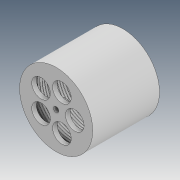
# Autodesk Inventor part: PeepCover
Saved by Autodesk Inventor 2020 (Build 240168000, 168)
## iProperties
Created: 2020-04-09
Part Number: PeepCover
Material: Generic
Document SubType Name: Modeling
Designer: Theo Cominotto
Density: 1 g/cm^3
Appearance: Default
Author: Theo Cominotto
Autodesk Inventor part; units mm, degrees
ref_plane "YZ Plane" through (0, 0, 0) normal (1, 0, 0) x (0, 1, 0)
ref_plane "XZ Plane" through (0, 0, 0) normal (0, 1, 0) x (-1, 0, 0)
ref_plane "XY Plane" through (0, 0, 0) normal (0, 0, 1) x (1, 0, 0)
sketch "Sketch1" plane through (0, 0, 0) normal (0, 0, 1) x (1, 0, 0)
  circle A0 centre (0, 0) radius 21.95
  circle A1 centre (0, 0) radius 23.55
  dimension "d0" = 43.9
  dimension "d1" = 1.6
  constraints: 2 centre point, 1 coincident
  measures "d0" diameter of A0
  measures "d1" radial gap between concentric circles of A0 A1
extrude "Extrusion1" add sketch "Sketch1" along normal blind 40
sketch "Sketch2" plane through (0, 0, 0) normal (0, 1, 0) x (-1, 0, 0)
  line L0 (23.55, 0) -> (-23.55, 0) projected
  line L1 (23.55, 0) -> (23.55, -1.2)
  line L2 (23.55, -0.6) -> (24.35, -0.6) construction
  line L3 (24.35, -0.6) -> (23.55, -1.2)
  line L4 (24.35, -0.6) -> (23.55, 0)
  line L5 (23.55, 0) -> (21.95, 0) construction
  line L6 (21.95, 40) -> (21.95, 0) construction
  line L7 (22.75, 0) -> (22.75, -1.2) construction
  line L8 (21.95, 0) -> (21.95, -1.2)
  line L9 (21.95, -0.6) -> (21.15, -0.6) construction
  line L10 (21.15, -0.6) -> (21.95, -1.2)
  line L11 (21.15, -0.6) -> (21.95, 0)
  point P0 (0, 0)
  dimension "d4" = 1.2
  dimension "d5" = 0.8
  constraints: 20 end point, 3 symmetric about line, 2 midpoint, 2 point on line, 2 vertical, 1 horizontal
  measures "d4" distance of L0.start L1.end
  measures "d5" distance of L2.start L2.end
coil "Coil1" sketch "Sketch2" operation add axis through (0, 0, -10) along (0, 0, 1) pitch 1.5 turns 26.666667 hand right contours L8 L10 L11
sketch "Sketch3" plane through (0, 0, 0) normal (0, 0, -1) x (-1, 0, 0)
  circle A0 centre (0, 0) radius 23.55 projected
extrude "Extrusion2" cut sketch "Sketch3" along normal blind 20
sketch "Sketch4" plane through (0, 0, 40) normal (0, 0, 1) x (1, 0, 0)
  circle A0 centre (0, 0) radius 23.55 projected
  line L0 (0, 0) -> (12, 0) construction
  circle A1 centre (12, 0) radius 6
  circle A2 centre (3.7082, 11.4127) radius 6
  circle A3 centre (-9.7082, 7.0534) radius 6
  circle A4 centre (-9.7082, -7.0534) radius 6
  circle A5 centre (3.7082, -11.4127) radius 6
  dimension "d16" = 12
  dimension "d17" = 12
  dimension "d20" = 360
  constraints: 5 centre point, 2 end point, 1 coincident, 1 horizontal, 11 other
  measures "d16" distance of L0.start L0.end
  measures "d17" diameter of A1
extrude "Extrusion3" add sketch "Sketch4" along normal blind 3
sketch "Sketch5" plane through (0, 0, 40) normal (0, 0, -1) x (-1, 0, 0)
  circle A0 centre (0, 0) radius 3.3
  dimension "d24" = 6.6
  constraints: 1 centre point, 1 coincident
  measures "d24" diameter of A0
extrude "Extrusion4" add sketch "Sketch5" along normal blind 4
chamfer "Chamfer1" distance 1 angle 45 1 edges at (3.3, 0, 36)
sketch "Sketch6" plane through (0, 0, 36) normal (0, 0, -1) x (-1, 0, 0)
  circle A0 centre (0, 0) radius 2.3 construction
  circle A1 centre (0, 0) radius 1.7
  dimension "d30" = 0.6
  constraints: 1 centre point
  measures "d30" radial gap between concentric circles of A0 A1
extrude "Extrusion5" cut sketch "Sketch6" against normal up to surface (7 mm away)
equation "\"d6\" = ThreadPitch"
equation "\"ThreadPitch\" = 1.5"
body "Solid1"
